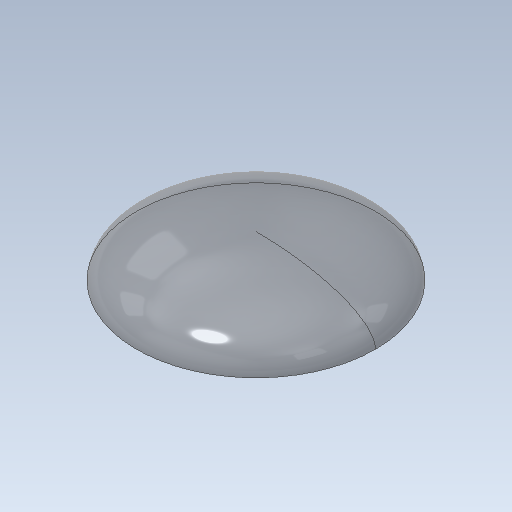
# Autodesk Inventor part: Manfrotto Logo 01 - 2
Saved by Autodesk Inventor 2020 (Build 240168000, 168)
## iProperties
Created: 2012-11-06
Part Number: Manfrotto Logo 01 - 2
Document SubType Name: Modeling
Designer: Lance
Density: 2.18 g/cm^3
Material: Glass
Mass: 0.123705 g
Surface Area: 1.26348 cm^2
Volume: 0.0567453 cm^3
Appearance: Light Gray
Author: Lance
Autodesk Inventor part; units mm, degrees
ref_plane "YZ Plane" through (0, 0, 0) normal (1, 0, 0) x (0, 1, 0)
ref_plane "XZ Plane" through (0, 0, 0) normal (0, 1, 0) x (-1, 0, 0)
ref_plane "XY Plane" through (0, 0, 0) normal (0, 0, 1) x (1, 0, 0)
sketch "Sketch4" plane through (0, 0, 0) normal (0, 0, 1) x (1, 0, 0)
  ellipse E0 centre (0, -0.75) end of major axis (4.25, -0.75) minor radius 1.5 (4.25, -0.75) -> (0, 0.75) ccw
  line L0 (0, -0.75) -> (0, 0.75)
  line L1 (0, -1.1605) -> (0, 1.713) projected
  line L2 (0, -0.75) -> (4.25, -0.75)
  point P0 (0, 0)
  dimension "d9" = 1.5
  dimension "d10" = 8.5
  constraints: 5 end point, 1 coincident, 1 collinear, 1 midpoint, 1 perpendicular, 1 vertical, 4 other
  measures "d9" distance from line of L0.end L2
  measures "d10" diameter of L2.end L1
revolve "Revolution1" add sketch "Sketch4" angle 360 about axis through (0, -0.75, 0) along (0, 1, 0)
body "Solid1"
